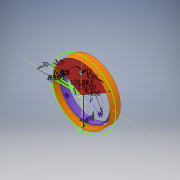
# Autodesk Inventor part: Baldachin
Saved by Autodesk Inventor 2018.2 (Build 222227000, 227)
## iProperties
Created: 2018-03-01
Part Number: Baldachin
Material: Generisch
Document SubType Name: Modeling
Designer: JochenAlt
Density: 1 g/cm^3
Appearance: Vorgabe
Author: JochenAlt
Autodesk Inventor part; units mm, degrees
ref_plane "YZ Plane" through (0, 0, 0) normal (1, 0, 0) x (0, 1, 0)
ref_plane "XZ Plane" through (0, 0, 0) normal (0, 1, 0) x (-1, 0, 0)
ref_plane "XY Plane" through (0, 0, 0) normal (0, 0, 1) x (1, 0, 0)
sketch "Skizze1" plane through (0, 0, 0) normal (0, 0, 1) x (1, 0, 0)
  line L0 (-87, 25.6288) -> (-85, 25.6288)
  line L1 (-85, 25.6288) -> (-85, -4.1591)
  line L2 (-87, -6.1591) -> (-87, 25.6288)
  line L3 (-87, -6.1591) -> (-85, -4.1591)
  line L4 (-190.6104, 0) -> (190.6104, 0) construction
  line L5 (-86.7879, -6.3712) -> (-84.7879, -4.3712)
  line L6 (-86.7879, -6.7712) -> (0, -6.7712)
  line L7 (-84.7879, -4.3712) -> (0, -4.3712)
  line L8 (-85, -4.1591) -> (-84.7879, -4.3712) construction
  line L9 (-87, -6.1591) -> (-86.7879, -6.3712) construction
  line L10 (-86.7879, -6.3712) -> (-86.7879, -6.7712)
  line L11 (-78, 25.6288) -> (-78, 7.6288)
  line L12 (-76.64, 4.2009) -> (-75.2247, 5.6162)
  line L13 (-76, 7.6288) -> (-76, 25.6288)
  line L14 (-78, 25.6288) -> (-76, 25.6288)
  line L15 (-76.4279, 3.9888) -> (-75.0126, 5.4041)
  line L16 (-85, -4.1591) -> (-84.7879, -4.3712) construction
  line L17 (-73, 4.6288) -> (0, 4.6288)
  line L18 (-73, 2.6288) -> (0, 2.6288)
  line L19 (0, 55.1351) -> (0, -17.0889) construction
  line L20 (0, 4.6288) -> (0, 2.6288)
  line L21 (0, -4.3712) -> (0, -6.7712)
  line L22 (-84.8939, -4.2651) -> (-52.2199, 28.4089) construction
  arc A0 (-78, 7.6288) -> (-73, 2.6288) centre (-73, 7.6288) ccw
  arc A1 (-76, 7.6288) -> (-73, 4.6288) centre (-73, 7.6288) ccw
  line L23 (-85, 25.9288) -> (-87.3, 25.9288)
  line L24 (-87.3, 25.9288) -> (-87.3, 24.37)
  line L25 (-88.8854, 25.2853) -> (-118.9659, 42.6523)
  line L26 (-118.9659, 42.6523) -> (-117.7159, 44.8173)
  line L27 (-117.7159, 44.8173) -> (-85, 25.9288)
  line L28 (-85, 25.9288) -> (-85, 25.9288)
  line L29 (-117.7159, 44.8173) -> (-74.1146, 44.8173)
  line L30 (-85, 25.6288) -> (-78, 25.6288) construction
  line L31 (-81.5, 25.6288) -> (-81.5, 44.8173) construction
  line L32 (0, -17.0889) -> (0, 55.1351) projected
  line L33 (-85, 25.9288) -> (-78, 25.9288)
  line L34 (-88.8854, 25.2853) -> (-88.8854, 18.6784)
  line L35 (-88.8854, 18.6784) -> (-87.3, 18.6784)
  line L36 (-87.3, 18.6784) -> (-87.3, 24.37)
  line L37 (-75.7, 18.6784) -> (-74.1146, 18.6784)
  line L38 (-74.1146, 18.6784) -> (-74.1146, 44.8173)
  line L39 (-78, 25.9288) -> (-78, 44.8173)
  line L40 (-78, 25.9288) -> (-75.7, 25.9288)
  line L41 (-75.7, 25.9288) -> (-75.7, 18.6784)
  point P0 (0, 0)
  point P1 (-75.7, 24.37)
  point P2 (-75.7, 24.37)
  dimension "d1" = 45
  dimension "d2" = 2
  dimension "d4" = 0.3
  dimension "d5" = 2.4
  dimension "d6" = 30
  dimension "d10" = 7
  dimension "d14" = 85
  dimension "d34" = 5
  dimension "d35" = 0.3
  dimension "d36" = 0.3
  dimension "d40" = 2.5
  constraints: 79 end point, 12 horizontal, 11 collinear, 9 perpendicular, 8 point on circle, 7 vertical, 6 parallel, 5 point on line, 4 tangent, 3 coincident, 3 midpoint, 2 centre point, 1 symmetric about line, 7 other
  measures "d1" angle of L3 L2
  measures "d2" distance between parallel lines of L1 L2
  measures "d4" distance between parallel lines of L5 L3
  measures "d5" distance between parallel lines of L6 L7
  measures "d6" distance between parallel lines of L0 L7
  measures "d10" distance between parallel lines of L11 L1
  measures "d14" distance between parallel lines of L19 L1
  measures "d34" radius of A0
  measures "d35" distance between parallel lines of L23 L0
  measures "d36" distance between parallel lines of L2 L24
  measures "d40" distance between parallel lines of L27 L25
revolve "Umdrehung1" add sketch "Skizze1" angle 360 about axis through (0, 0, 0) along (0, -1, 0) contours L5 L7 L21 L6 L10
revolve "Umdrehung2" add sketch "Skizze1" angle 360 about axis through (0, 0, 0) along (0, -1, 0) separate body contours L0 L1 L3 L2
revolve "Umdrehung3" add sketch "Skizze1" angle 360 about axis through (0, 0, 0) along (0, -1, 0) separate body contours L14 L13 A1 L12 A0 L11
revolve "Umdrehung4" add sketch "Skizze1" angle 360 about axis through (0, 0, 0) along (0, -1, 0) separate body contours L15 A1 L17 L20 L18 A0
sketch "Skizze2" plane through (0, 0, 0) normal (1, 0, 0) x (0, 1, 0)
  circle A0 centre (11.1288, 0) radius 2.15
  line L0 (25.6288, -76) -> (25.6288, 76) construction
  line L1 (-4.3712, 84.7879) -> (-4.3712, -84.7879) construction
  line L2 (-13.8156, 6) -> (-13.8156, -6) construction
  line L3 (25.6288, -76) -> (25.6288, 76) construction
  line L4 (-4.1591, 85) -> (-4.1591, -85) construction
  line L5 (25.6288, 85) -> (25.6288, -85) construction
  line L6 (-6.3712, 86.7879) -> (-6.3712, -86.7879) construction
  line L7 (-4.3712, 84.7879) -> (-4.3712, -84.7879) construction
  line L8 (-6.7712, 86.7879) -> (-6.7712, -86.7879) construction
  line L9 (-22.6956, 0) -> (22.6644, 0) construction
  point P0 (0, 0)
  dimension "d15" = 4.3
  dimension "d45" = 14.5
  constraints: 1 centre point, 1 point on line, 1 other
  measures "d15" diameter of A0
  measures "d45" distance from line of A0.centre L0
extrude "Extrusion1" cut sketch "Skizze2" along normal through all both and the other way through all bodies 3
extrude "Extrusion2" cut sketch "Skizze2" along normal through all both and the other way through all bodies 2
sketch "Skizze3" plane through (0, 0, 0) normal (1, 0, 0) x (0, 1, 0)
  line L0 (37.3251, -96.6554) -> (-18.7979, -96.6554)
  line L1 (-18.7979, -96.6554) -> (-18.7979, -82.3534)
  line L2 (-18.7979, -82.3534) -> (37.3251, -82.3534)
  line L3 (37.3251, -82.3534) -> (37.3251, -96.6554)
  line L4 (25.6288, -76) -> (7.6288, -76) projected
  line L5 (5.6162, -76) -> (25.6288, -76)
  line L6 (25.6288, -76) -> (25.6288, -72)
  line L7 (25.6288, -72) -> (5.6162, -72)
  line L8 (5.6162, -72) -> (5.6162, -76)
  line L9 (7.6288, -78) -> (25.6288, -78) projected
  line L10 (25.6288, -78) -> (3.0772, -78)
  line L11 (3.0772, -78) -> (3.0772, -73.7)
  line L12 (3.0772, -73.7) -> (25.6288, -73.7)
  line L13 (25.6288, -73.7) -> (25.6288, -78)
  line L14 (5.6162, -75.2247) -> (5.6162, 75.2247) construction
  point P0 (0, 0)
  dimension "d26" = 4
  dimension "d32" = 4.3
  constraints: 24 end point, 6 parallel, 5 point on line, 3 horizontal, 3 perpendicular
  measures "d26" distance between parallel lines of L7 L4
  measures "d32" distance between parallel lines of L12 L10
extrude "Extrusion3" cut sketch "Skizze3" along normal mid plane 0.2 contours L0 L1 L2 L3 bodies 2
extrude "Extrusion5" add sketch "Skizze3" along normal mid plane 8 contours L4 L5 L8 L12 L6 | L12 L8 L7 L6 bodies 3
extrude "Extrusion6" cut sketch "Skizze3" along normal mid plane 4.3 contours L13 L9 L10 L11 L12 L8 L5 L4 | L4 L5 L8 L12 L6 bodies 3
extrude "Extrusion4" cut sketch "Skizze3" along normal mid plane 2 bodies 3
revolve "Umdrehung6" add sketch "Skizze1" angle 30 mid plane about axis through (0, -10, 0) along (0, 1, 0) separate body contours L23 L24 L36 L35 L34 L25 L26 L27 | L27 L29 L39 L33 | L39 L29 L38 L37 L41 L40
revolve "Umdrehung8" cut sketch "Skizze1" angle 26 mid plane about axis through (0, 0, 0) along (0, -1, 0) contours L27 L29 L39 L33
sketch "Skizze4" plane through (0, 0, 0) normal (0, 1, 0) x (-1, 0, 0)
  circle A0 centre (0, 0) radius 57.735 construction
  circle A1 centre (0, 57.735) radius 6
  line L0 (0, 0) -> (-50, -28.8675) construction
  line L1 (0, 0) -> (50, -28.8675) construction
  line L2 (0, 0) -> (0, 57.735) construction
  circle A2 centre (-50, -28.8675) radius 6
  circle A3 centre (50, -28.8675) radius 6
  line L3 (0, 0) -> (0, -98.0914)
  line L4 (0, 0) -> (84.9497, 49.0457)
  line L5 (0, 0) -> (-84.9497, 49.0457)
  circle A4 centre (0, 0) radius 98.0914
  dimension "d51" = 12
  dimension "d52" = 120
  dimension "d53" = 120
  dimension "d59" = 100
  constraints: 12 end point, 6 point on circle, 5 centre point, 4 coincident, 2 collinear, 2 equal radius, 2 vertical
  measures "d51" diameter of A1
  measures "d52" angle of L1 L2
  measures "d53" angle of L0 L2
  measures "d59" distance of L0.end L2.end
extrude "Extrusion7" cut sketch "Skizze4" against normal through all contours A1 | A2 | A3 bodies 4 1
extrude "Extrusion8" cut sketch "Skizze4" along normal through all both and the other way through all contours A1 | A2 | A3 bodies 4
extrude "Extrusion9" cut sketch "Skizze4" against normal blind 10 contours L5 A4 L4 keep common part bodies 1
extrude "Extrusion10" cut sketch "Skizze4" along normal blind 10 contours L5 A4 L4 keep common part bodies 4
equation "\"d36\" = d35"
